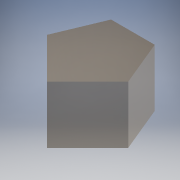
# Autodesk Inventor part: Prisma-90
Saved by Autodesk Inventor 2017 (Build 210142000, 142)
## iProperties
Created: 2017-08-01
Part Number: Prisma-90
Material: Glass
Document SubType Name: Modeling
Designer: vmiguel
Density: 2.18 g/cm^3
Appearance: Polycarbonate - Smoked
Author: vmiguel
Autodesk Inventor part; units mm, degrees
ref_plane "YZ Plane" through (0, 0, 0) normal (1, 0, 0) x (0, 1, 0)
ref_plane "XZ Plane" through (0, 0, 0) normal (0, 1, 0) x (-1, 0, 0)
ref_plane "XY Plane" through (0, 0, 0) normal (0, 0, 1) x (1, 0, 0)
sketch "Sketch1" plane through (0, 0, 0) normal (0, 0, 1) x (1, 0, 0)
  line L0 (5.3033, -5.3033) -> (0, 0) construction
  line L1 (0, 0) -> (-5.3033, -5.3033) construction
  line L2 (0, -10.6066) -> (10.6066, 0)
  line L3 (10.6066, 0) -> (5.7063, 11.8303)
  line L4 (5.7063, 11.8303) -> (-5.7063, 11.8303)
  line L5 (-5.7063, 11.8303) -> (-10.6066, 0)
  line L6 (-10.6066, 0) -> (0, -10.6066)
  line L7 (0, -10.6066) -> (0, 11.8303) construction
  dimension "d0" = 90
  dimension "d1" = 112.5
  dimension "d2" = 112.5
  dimension "d3" = 112.5
  dimension "d4" = 15
  dimension "d5" = 12.805
  constraints: 16 end point, 4 perpendicular, 3 midpoint, 1 coincident, 1 horizontal
  measures "d0" angle of L6 L2
  measures "d1" angle of L3 L2
  measures "d2" angle of L3 L4
  measures "d3" angle of L6 L5
  measures "d4" distance of L2.start L2.end
  measures "d5" distance of L2.end L3.end
extrude "Extrusion1" add sketch "Sketch1" along normal blind 15
equation "\"d2\" = d1"
equation "\"d3\" = d1"
body "Solid1"
